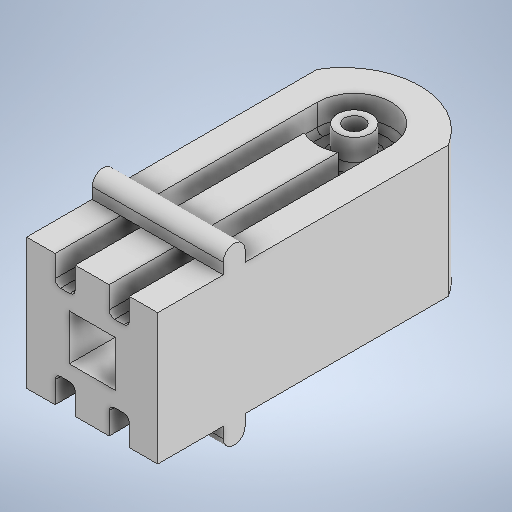
# Autodesk Inventor part: Nedre del av kne proto1
Saved by Autodesk Inventor 2025.1 (Build 291241020, 241B)
## iProperties
Created: 2024-10-03
Part Number: Nedre del av kne proto1
Material: Generic
Document SubType Name: Modeling
Designer: morte
Density: 1 g/cm^3
Appearance: Default
Author: morte
Autodesk Inventor part; units mm, degrees
ref_plane "YZ Plane" through (0, 0, 0) normal (1, 0, 0) x (0, 1, 0)
ref_plane "XY Plane" through (0, 0, 0) normal (0, 0, 1) x (1, 0, 0)
sketch "Sketch1" plane through (0, 0, 0) normal (0, 0, 1) x (1, 0, 0)
  line L0 (-2.1, -2.1) -> (2.1, -2.1)
  line L1 (2.1, -2.1) -> (2.1, 2.1)
  line L2 (2.1, 2.1) -> (-2.1, 2.1)
  line L3 (-2.1, 2.1) -> (-2.1, -2.1)
  line L4 (-2.1, -2.1) -> (2.1, 2.1) construction
  line L5 (2.1, -2.1) -> (-2.1, 2.1) construction
  line L6 (-6, -6) -> (6, -6)
  line L7 (6, -6) -> (6, 6)
  line L8 (6, 6) -> (-6, 6)
  line L9 (-6, 6) -> (-6, -6)
  line L10 (-6, -6) -> (6, 6) construction
  line L11 (6, -6) -> (-6, 6) construction
  line L12 (0, 6) -> (0, 2.1)
  point P0 (0, 0)
  dimension "d0" = 4.2
  dimension "d1" = 4.2
  dimension "d2" = 12
  dimension "d3" = 12
  dimension "d93" = 3.9
  constraints: 26 end point, 6 midpoint, 4 parallel, 2 horizontal, 2 perpendicular, 1 point on line
  measures "d0" distance of L1.end L2.end
  measures "d1" distance of L0.end L1.end
  measures "d2" distance of L8.end L6.start
  measures "d3" distance of L7.end L8.end
  measures "d93" distance of L12.start L12.end
extrude "Extrusion1" add sketch "Sketch1" along normal mid plane 30
sketch "Sketch2" plane through (-6, 6, 15) normal (0, 1, 0) x (1, 0, 0)
  line L0 (0, 30) -> (0, 0) projected
  line L1 (0, 0) -> (0, 6)
  line L2 (0, 0) -> (0, 8)
  line L3 (0, 6) -> (12, 6)
  line L4 (12, 30) -> (12, 0) projected
  line L5 (0, 8) -> (12, 8)
  line L6 (12, 6) -> (12, 8)
  point P0 (6, 15)
  dimension "d6" = 6
  dimension "d7" = 8
  dimension "d8" = 2
  constraints: 10 end point, 3 point on line, 2 horizontal, 1 collinear
  measures "d6" distance of L0.end L1.end
  measures "d7" distance of L0.end L2.end
  measures "d8" distance of L3.end L5.end
extrude "Extrusion2" add sketch "Sketch2" along normal blind 2
sketch "Sketch3" plane through (-6, 6, -15) normal (0, 1, 0) x (1, 0, 0)
  line L0 (0, 0) -> (0, -30) projected
  line L1 (12, -30) -> (12, 0) projected
  line L2 (0, 0) -> (0, -22) projected
  line L3 (12, -30) -> (0, -30) projected
  line L4 (9.1, -31) -> (2.9, -31)
  line L5 (6, -6) -> (6, 0)
  circle A0 centre (6, -6) radius 1.55
  line L6 (2.8, -31) -> (4, -31)
  line L7 (9.2, -31) -> (8, -31)
  circle A1 centre (6, -6) radius 3.4
  line L8 (2.6, -6) -> (2.6, -31)
  line L9 (2.6, -6) -> (27.6, -6) construction
  line L10 (2.6, -31) -> (4, -31)
  line L11 (9.4, -6) -> (9.4, -31)
  line L12 (9.4, -6) -> (34.4, -6) construction
  line L13 (9.4, -31) -> (8, -31)
  line L14 (4.45, -6) -> (4.45, -31)
  line L15 (4.45, -6) -> (29.45, -6) construction
  line L16 (7.55, -6) -> (7.55, -31)
  line L17 (7.55, -6) -> (32.55, -6) construction
  point P0 (6, -15)
  point P1 (9.4, -30)
  point P2 (2.6, -30)
  point P3 (4.45, -30)
  point P4 (4.45, -9.0261)
  point P5 (7.55, -9.0261)
  point P6 (7.55, -30)
  dimension "d139" = 6
  dimension "d145" = 3.1
  dimension "d183" = 6.8
  dimension "d184" = 90
  dimension "d185" = 90
  dimension "d190" = 90
  dimension "d191" = 90
  dimension "d204" = 6
  constraints: 28 end point, 6 point on line, 5 horizontal, 4 perpendicular, 4 point on circle, 3 collinear, 2 centre point, 1 coincident, 1 tangent
  measures "d139" distance of L5.start L5.end
  measures "d145" diameter of A0
  measures "d183" diameter of A1
  measures "d184" angle of L8 L9
  measures "d185" angle of L11 L12
  measures "d190" angle of L14 L15
  measures "d191" angle of L16 L17
  measures "d204" horizontal distance of L0.start A0.centre
extrude "Extrusion3" cut sketch "Sketch3" against normal blind 2.5 contours L3 L16 A1 L11 | A1 L16 A0 L5 | L3 L8 A1 L14 | A1 L14 A0 L16 | L5 A0 L14 A1
ref_plane "Work Plane3" through (0, -6, 0) normal (0, 1, 0) x (-1, 0, 0)
sketch "Sketch16" plane through (-6, -6, -15) normal (0, -1, 0) x (1, 0, 0)
  line L0 (12, 0) -> (0, 0) projected
  line L1 (0, 0) -> (6, 0)
  line L2 (6, 0) -> (6, 6)
  circle A0 centre (6, 6) radius 1.55
  arc A1 (7.55, 6) -> (7.55, 6) centre (6, 6) ccw projected
  line L3 (10.2, 6) -> (36.7126, 6) construction
  line L4 (8.95, 32.5126) -> (7.75, 32.5126)
  line L5 (2.8, 6) -> (29.3126, 6) construction
  line L6 (7.55, 6) -> (9.4, 6)
  circle A2 centre (6, 6) radius 3.4
  line L7 (9.4, 6) -> (9.4, 32.5126)
  line L8 (9.4, 6) -> (35.9126, 6) construction
  line L9 (9.4, 32.5126) -> (7.75, 32.5126)
  line L10 (2.6, 6) -> (2.6, 32.5126)
  line L11 (2.6, 6) -> (29.1126, 6) construction
  line L12 (7.55, 6) -> (7.55, 32.5126)
  line L13 (7.55, 6) -> (34.0626, 6) construction
  line L14 (7.55, 32.5126) -> (9.4, 32.5126)
  line L15 (4.45, 6) -> (4.45, 32.5126)
  line L16 (4.45, 6) -> (30.9626, 6) construction
  line L17 (4.45, 32.5126) -> (2.6, 32.5126)
  point P0 (10.1, 6)
  point P1 (4.45, 9.0261)
  point P2 (7.55, 9.0261)
  dimension "d155" = 6
  dimension "d156" = 6
  dimension "d181" = 90
  dimension "d182" = 90
  dimension "d187" = 3.1
  dimension "d188" = 90
  dimension "d189" = 90
  dimension "d198" = 6.8
  constraints: 34 end point, 8 horizontal, 5 perpendicular, 4 point on circle, 3 point on line, 2 centre point, 2 coincident, 2 collinear, 1 midpoint, 1 tangent
  measures "d155" distance of L0.end L1.end
  measures "d156" distance of L1.end L2.end
  measures "d181" angle of L8 L7
  measures "d182" angle of L11 L10
  measures "d187" diameter of A0
  measures "d188" angle of L13 L12
  measures "d189" angle of L16 L15
  measures "d198" diameter of A2
extrude "Extrusion12" cut sketch "Sketch16" against normal blind 2.5 contours A2 L15 A0 L2 | L2 A0 L6 A2 | L10 L17 L15 A2 | L6 L12 A2 | A2 L12 L14 L4 L9 L7 | L15 A2 L12 A0
sketch "Sketch17" plane through (0, -6, -9) normal (0, -1, 0) x (1, 0, 0)
  circle A0 centre (0, 0) radius 0.9
  point P0 (0, 9)
  point P1 (3.1, 0)
  dimension "d186" = 1.8
  constraints: 1 centre point, 1 coincident
  measures "d186" diameter of A0
extrude "Extrusion13" cut sketch "Sketch17" against normal through all
sketch "Sketch18" plane through (0, -6, -9) normal (0, -1, 0) x (1, 0, 0)
  line L0 (0, 0) -> (0, 1)
  arc A0 (-7, 1) -> (7, 1) centre (0, 1) ccw
  line L1 (0, 1) -> (7, 1)
  line L2 (0, 1) -> (-7, 1)
  line L3 (7, 1) -> (7, -9.6793)
  line L4 (7, -9.6793) -> (-7, -9.6793)
  line L5 (-7, -9.6793) -> (-7, 1)
  point P0 (0, 9)
  dimension "d167" = 1
  constraints: 12 end point, 2 perpendicular, 2 point on circle, 2 vertical, 1 centre point, 1 coincident, 1 horizontal, 1 point on line
  measures "d167" distance of L0.start L0.end
extrude "Extrusion14" cut sketch "Sketch18" against normal through all contours A0 L3 L4 L5
fillet "Fillet11" radius 1 2 edges at (0, 8, 7) (0, 8, 9)
fillet "Fillet12" radius 0.5 12 edges at (3.4, 3.5, 3) (-3.4, 3.5, 3) (0, 3.5, -12.4) (-1.55, 3.5, -9) (1.55, 3.5, 4.5131) (-1.55, 3.5, 4.5131) (0, -3.5, -12.4) (3.4, -3.5, 3) (-3.4, -3.5, 3) (-1.55, -3.5, -9) (1.55, -3.5, 4.5131) (-1.55, -3.5, 4.5131)
sketch "Sketch19" plane through (0, -6, -9) normal (0, -1, 0) x (1, 0, 0)
  line L0 (0, 0) -> (0, 24)
  line L1 (1.55, 24) -> (-1.55, 24) projected
  line L2 (3.4, 24) -> (6, 24) projected
  line L3 (0, 24) -> (6, 24)
  line L4 (6, 24) -> (6, 18)
  line L5 (3.4, 16) -> (6, 16) projected
  line L6 (-6, 16) -> (-3.4, 16) projected
  line L7 (6, 16) -> (-6, 16)
  line L8 (-6, 16) -> (-6, 18) projected
  line L9 (-6, 16) -> (-6, 18)
  line L10 (-6, 18) -> (6, 18)
  line L11 (6, 18) -> (6, 15.7444)
  point P0 (0, 9)
  point P1 (6, 16)
  point P2 (-3.4, 16)
  point P3 (3.4, 16)
  dimension "d194" = 6
  constraints: 14 end point, 2 collinear, 1 horizontal, 1 midpoint, 1 perpendicular, 1 vertical
  measures "d194" distance of L2.end L4.end
extrude "Extrusion15" add sketch "Sketch19" along normal blind 2 contours L7 L6 L8 L10 L0 | L0 L10 L11 L5 L7
fillet "Fillet13" radius 1 2 edges at (0, -8, 7) (0, -8, 9)
body "Solid1"
